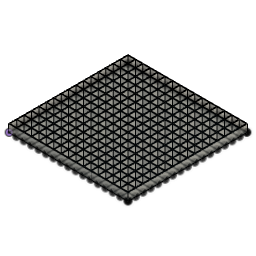
WLED Cube 16x16 Spacer v4 (Autodesk Fusion 360 design; units mm, degrees)
Autodesk Fusion 360 part; units mm, degrees
sketch "Sketch1" plane through (0, 0, 0) normal (0, 0, 1) x (1, 0, 0)
  line L0 (0, 0) -> (160, 0)
  line L1 (0, 0) -> (0, 160)
  line L2 (10, 0) -> (10, 160)
  line L3 (20, 0) -> (20, 160)
  line L4 (30, 0) -> (30, 160)
  line L5 (40, 0) -> (40, 160)
  line L6 (50, 0) -> (50, 160)
  line L7 (60, 0) -> (60, 160)
  line L8 (70, 0) -> (70, 160)
  line L9 (80, 0) -> (80, 160)
  line L10 (90, 0) -> (90, 160)
  line L11 (100, 0) -> (100, 160)
  line L12 (110, 0) -> (110, 160)
  line L13 (120, 0) -> (120, 160)
  line L14 (130, 0) -> (130, 160)
  line L15 (140, 0) -> (140, 160)
  line L16 (150, 0) -> (150, 160)
  line L17 (160, 0) -> (160, 160)
  line L18 (0, 10) -> (160, 10)
  line L19 (0, 20) -> (160, 20)
  line L20 (0, 30) -> (160, 30)
  line L21 (0, 40) -> (160, 40)
  line L22 (0, 50) -> (160, 50)
  line L23 (0, 60) -> (160, 60)
  line L24 (0, 70) -> (160, 70)
  line L25 (0, 80) -> (160, 80)
  line L26 (0, 90) -> (160, 90)
  line L27 (0, 100) -> (160, 100)
  line L28 (0, 110) -> (160, 110)
  line L29 (0, 120) -> (160, 120)
  line L30 (0, 130) -> (160, 130)
  line L31 (0, 140) -> (160, 140)
  line L32 (0, 150) -> (160, 150)
  line L33 (0, 160) -> (160, 160)
  dimension "d1" = 160
  dimension "d2" = 160
  dimension "d5" = 10
  dimension "d6" = 0
  dimension "d9" = 0
  dimension "d10" = 10
  constraint coincident L0.start L1.start
  constraint horizontal L0
  constraint perpendicular L0 L1
  measures "d1" distance of L0.start L0.end
  measures "d2" distance of L0.start L1.end
extrude "Extrude1" add sketch "Sketch1" along normal blind 2 thin wall 1 centred open curves L1 makes body 1
extrude "Extrude2" add sketch "Sketch1" along normal blind 1.5 thin wall 1 centred separate body open curves L0 makes body 2
pattern_linear "R-Pattern1" count 17 spacing 10 along (0, 1, 0) of bodies 2 makes body 3 at (53.3333, 10.5, 0.5) makes body 4 at (53.3333, 20.5, 0.5) makes body 5 at (53.3333, 30.5, 0.5) makes body 6 at (53.3333, 40.5, 0.5) makes body 7 at (53.3333, 50.5, 0.5) makes body 8 at (53.3333, 60.5, 0.5) makes body 9 at (53.3333, 70.5, 0.5) makes body 10 at (53.3333, 80.5, 0.5) makes body 11 at (53.3333, 90.5, 0.5) makes body 12 at (53.3333, 100.5, 0.5) makes body 13 at (53.3333, 110.5, 0.5) makes body 14 at (53.3333, 120.5, 0.5) makes body 15 at (53.3333, 130.5, 0.5) makes body 16 at (53.3333, 140.5, 0.5) makes body 17 at (53.3333, 150.5, 0.5) makes body 18 at (53.3333, 160.5, 0.5)
pattern_linear "R-Pattern2" count 17 spacing 10 along (1, 0, 0) of bodies 1 makes body 19 at (9.5, 53.3333, 1.3333) makes body 20 at (19.5, 53.3333, 1.3333) makes body 21 at (29.5, 53.3333, 1.3333) makes body 22 at (39.5, 53.3333, 1.3333) makes body 23 at (49.5, 53.3333, 1.3333) makes body 24 at (59.5, 53.3333, 1.3333) makes body 25 at (69.5, 53.3333, 1.3333) makes body 26 at (79.5, 53.3333, 1.3333) makes body 27 at (89.5, 53.3333, 1.3333) makes body 28 at (99.5, 53.3333, 1.3333) makes body 29 at (109.5, 53.3333, 1.3333) makes body 30 at (119.5, 53.3333, 1.3333) makes body 31 at (129.5, 53.3333, 1.3333) makes body 32 at (139.5, 53.3333, 1.3333) makes body 33 at (149.5, 53.3333, 1.3333) makes body 34 at (159.5, 53.3333, 1.3333)
extrude "Extrude3" add 1 faces at (53.3333, 40.1667, 1.5) along direction (0, 0, 1) blind 0.5 on bodies 6 bodies 1 2 3 4 5 7 8 9 10 11 12 13 14 15 16 17 18 6 19 20 21 22 23 24 25 26 27 28 29 30 31 32 33 34
extrude "Extrude4" add 1 faces at (53.3333, 30.1667, 1.5) along direction (0, 0, 1) blind 0.5 on bodies 5 bodies 1 2 3 4 7 8 9 10 11 12 13 14 15 16 17 18 5
extrude "Extrude5" add 1 faces at (53.3333, 50.1667, 1.5) along direction (0, 0, 1) blind 0.5 on bodies 7 bodies 1 2 3 4 8 9 10 11 12 13 14 15 16 17 18 7
extrude "Extrude6" add 3 faces at (53.3333, 60.1667, 1.5) (53.3333, 70.1667, 1.5) (53.3333, 80.1667, 1.5) along direction (0, 0, 1) blind 0.5 on bodies 8 9 10 bodies 1 2 3 4 11 12 13 14 15 16 17 18 8 9 10
extrude "Extrude7" add 8 faces at (53.3333, 90.1667, 1.5) (53.3333, 100.1667, 1.5) (53.3333, 110.1667, 1.5) (53.3333, 120.1667, 1.5) (53.3333, 130.1667, 1.5) (53.3333, 140.1667, 1.5) (53.3333, 150.1667, 1.5) (53.3333, 160.1667, 1.5) along direction (0, 0, 1) blind 0.5 on bodies 11 12 13 14 15 16 17 18 bodies 1 2 3 4 11 12 13 14 15 16 17 18
extrude "Extrude8" add 3 faces at (53.3333, 20.1667, 1.5) (53.3333, 10.1667, 1.5) (53.3333, 0.1667, 1.5) along direction (0, 0, 1) blind 0.5 on bodies 2 3 4 bodies 1 4 2 3
box "BoxPrimitive1" add length 2 width 0.5 height 0.5 placed x (0, 0, -1) y (1, 0, 0) z (0, -1, 0) at (-0.5, 0, 2) bodies 1
box "BoxPrimitive2" add length 2 width 0.5 height 0.5 placed x (0, 0, -1) y (0, -1, 0) z (-1, 0, 0) at (0, 160.5, 2) bodies 1
box "BoxPrimitive3" add length 2 width 0.5 height 0.5 placed x (0, 0, -1) y (0, 1, 0) z (1, 0, 0) at (160, -0.5, 2) bodies 1
sketch "Sketch5" plane through (0, 0, 0) normal (0, 0, 1) x (1, 0, 0)
box "BoxPrimitive4" add length 2 width 0.5 height 0.5 placed x (0, 0, -1) y (-1, 0, 0) z (0, 1, 0) at (160.5, 160, 2) bodies 1
extrude "Extrude9" add 1 faces at (-0.1667, 96.8333, 2) along direction (0, 0, 1) blind 8.2 on bodies 1 bodies 1
